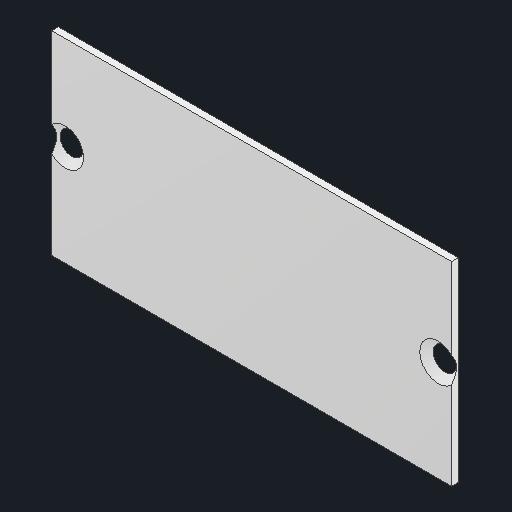
# Autodesk Inventor part: back
Saved by Autodesk Inventor 2023 (Build 270158000, 158)
## iProperties
Created: 2024-05-26
Part Number: back
Material: ABS Plastic
Document SubType Name: Modeling
Designer: szymo
Density: 1.06 g/cm^3
Appearance: Smooth - White
Mass: 1.79903 g
Surface Area: 36.0196 cm^2
Volume: 1.6972 cm^3
Author: szymo
Autodesk Inventor part; units mm, degrees
ref_plane "YZ Plane" through (0, 0, 0) normal (1, 0, 0) x (0, 1, 0)
ref_plane "XZ Plane" through (0, 0, 0) normal (0, 1, 0) x (-1, 0, 0)
ref_plane "XY Plane" through (0, 0, 0) normal (0, 0, 1) x (1, 0, 0)
sketch "Sketch1" plane through (0, 0, 0) normal (0, 0, 1) x (1, 0, 0)
  circle A0 centre (-20.8, 15) radius 1.75 projected
  arc A1 (-18.8, 17.2679) -> (-19.3, 18.134) centre (-19.8, 17.2679) ccw projected
  arc A2 (-19.8, 19) -> (-19.3, 18.134) centre (-18.8, 19) ccw projected
  line L0 (-19.8, 19) -> (-19.8, 29) projected
  line L1 (-22.8, 29) -> (-19.8, 29) projected
  line L2 (-22.8, 25.5) -> (-22.8, 29) projected
  line L3 (-22.8, 0) -> (-22.8, 25.5) projected
  line L4 (-22.8, 0) -> (-17.8, 0) projected
  line L5 (-17.8, 0) -> (-17.8, 8) projected
  line L6 (-19.8, 8) -> (-17.8, 8) projected
  line L7 (-19.8, 8) -> (-19.8, 11) projected
  arc A3 (-19.3, 11.866) -> (-19.8, 11) centre (-18.8, 11) ccw projected
  arc A4 (-19.3, 11.866) -> (-18.8, 12.7321) centre (-19.8, 12.7321) ccw projected
  line L8 (-18.8, 12.7321) -> (-18.8, 17.2679) projected
  circle A5 centre (34.8, 15) radius 1.75 projected
  arc A6 (33.3, 18.134) -> (32.8, 17.2679) centre (33.8, 17.2679) ccw projected
  line L9 (32.8, 12.7321) -> (32.8, 17.2679) projected
  arc A7 (32.8, 12.7321) -> (33.3, 11.866) centre (33.8, 12.7321) ccw projected
  arc A8 (33.8, 11) -> (33.3, 11.866) centre (32.8, 11) ccw projected
  line L10 (33.8, 8) -> (33.8, 11) projected
  line L11 (33.8, 8) -> (31.8, 8) projected
  line L12 (31.8, 0) -> (31.8, 8) projected
  line L13 (36.8, 0) -> (31.8, 0) projected
  line L14 (36.8, 0) -> (36.8, 25.5) projected
  line L15 (36.8, 25.5) -> (36.8, 29) projected
  line L16 (36.8, 29) -> (33.8, 29) projected
  line L17 (33.8, 19) -> (33.8, 29) projected
  arc A9 (33.3, 18.134) -> (33.8, 19) centre (32.8, 19) ccw projected
  line L18 (-22.8, 29) -> (36.8, 29)
  line L19 (36.8, 29) -> (36.8, 0)
  line L20 (36.8, 0) -> (-22.8, 0)
  line L21 (-22.8, 0) -> (-22.8, 29)
  point P0 (0, 0)
  constraints: 8 end point, 2 parallel, 1 horizontal, 1 perpendicular
extrude "Extrusion1" add sketch "Sketch1" along normal blind 1 contours A0 | L8 A4 A3 L7 L6 L5 L4 L3 L2 L1 L0 A2 A1 | A1 A2 L0 L18 L17 A9 A6 L9 A7 A8 L10 L11 L12 L20 L5 L6 L7 A3 A4 L8 | L16 L15 L14 L13 L12 L11 L10 A8 A7 L9 A6 A9 L17 | A5
sketch "Sketch2" plane through (0, 0, 1) normal (0, 0, 1) x (1, 0, 0)
  circle A0 centre (-20.8, 15) radius 1.75 projected
  circle A1 centre (34.8, 15) radius 1.75 projected
  point P0 (0, 0)
  constraints: 2 coincident
hole "Hole1" at (-20.8, 15, 1) at (34.8, 15, 1) direction (0, 0, -1) diameter 3.1 end through all countersink diameter 5.5 countersink angle 90 clearance for "Countersunk Flat Head Screw ISO 2009/7046" size "M2.5" standard "ISO"
body "Solid1"
